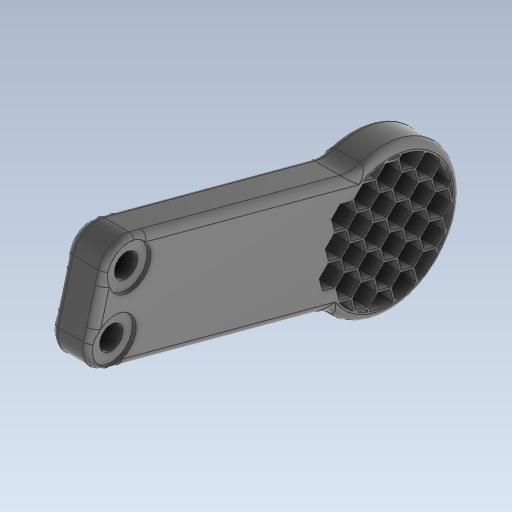
# Autodesk Inventor part: RearBumper
Saved by Autodesk Inventor 2020.4 (Build 244396000, 396)
## iProperties
Part Number: RearBumper
Material: PC/ABS プラスチック
Document SubType Name: Modeling
Designer: Masato Kubotera
Density: 0.357273 g/cm^3
Appearance: 滑らか - 黒
Description: TPU
Author: Masato Kubotera
Autodesk Inventor part; units mm, degrees
(part 1 of 2)
ref_plane "YZ Plane" through (0, 0, 0) normal (1, 0, 0) x (0, 1, 0)
ref_plane "XZ Plane" through (0, 0, 0) normal (0, 1, 0) x (-1, 0, 0)
ref_plane "XY Plane" through (0, 0, 0) normal (0, 0, 1) x (1, 0, 0)
derived "Trunk_basis.ipt"
sketch "スケッチ1" plane through (0, 0, 0) normal (0, 1, 0) x (-1, 0, 0)
  line L0 (0, 22) -> (0, -142.9) construction
  circle A0 centre (5, 0) radius 10.5 construction
  line L1 (-7, 16) -> (36, 16) construction
  line L2 (36, 16) -> (36, -16) construction
  line L3 (36, -16) -> (-7, -16) construction
  line L4 (-7, -16) -> (-7, 16) construction
  line L5 (-7, 16) -> (36, -16) construction
  line L6 (36, 16) -> (-7, -16) construction
  line L7 (33, 13.5) -> (6, 13.5) construction
  line L8 (6, 13.5) -> (6, -13.5) construction
  line L9 (6, -13.5) -> (33, -13.5) construction
  line L10 (33, -13.5) -> (33, 13.5) construction
  line L11 (33, 13.5) -> (6, -13.5) construction
  line L12 (6, 13.5) -> (33, -13.5) construction
  line L13 (-7, 0) -> (36, 0) construction
  arc A1 (5, 16) -> (-7, 10.583005) centre (5, 0) ccw construction
  line L14 (43.75, -16.25) -> (5, -16.25)
  line L15 (5, 16.25) -> (43.75, 16.25)
  line L16 (44.75, 15.25) -> (44.75, -15.25)
  arc A2 (5, 16.25) -> (-6.737613, 11.237924) centre (5, 0) ccw
  arc A3 (-6.737613, 11.237924) -> (-7.25, 9.917415) centre (-6.271109, 10.297247) ccw
  circle A4 centre (6, 13.5) radius 1.35
  line L17 (19.5, 13.5) -> (19.5, -13.5) construction
  circle A5 centre (33, 13.5) radius 1.35
  line L18 (-15, 22) -> (-20, 17)
  line L19 (-20, 17) -> (-20, -19)
  line L20 (-20, -19) -> (-28.5, -27.5)
  line L21 (-28.5, -27.5) -> (-28.5, -103)
  line L22 (57.5, -22.5) -> (57.5, 17)
  line L23 (57.5, 17) -> (52.5, 22)
  line L24 (52.5, 22) -> (-15, 22)
  line L25 (-35.55968, -116.552914) -> (-28.5, -142.9)
  line L26 (-16, -139) -> (-16, -94) construction
  line L27 (-7.5, -140.484924) -> (-7.5, -142.9)
  line L28 (-7.5, -142.9) -> (7.5, -142.9)
  line L29 (7.5, -140.484924) -> (7.5, -142.9)
  arc A6 (-7.5, -140.484924) -> (-8.984924, -139) centre (-8.242462, -139.742462) ccw
  line L30 (-17.5, -138.995456) -> (-17.5, -133) construction
  line L31 (-19, -133) -> (-16, -133) construction
  line L32 (-19, -133) -> (-19, -139) construction
  line L33 (-16, -133) -> (-16, -139) construction
  line L34 (-15, 22) -> (-10, 22) construction
  line L35 (-10, 22) -> (-10, -22) construction
  line L36 (-10, -22) -> (-15, -22) construction
  line L37 (-15, -22) -> (-15, 22) construction
  line L38 (-15, 22) -> (-10, -22) construction
  line L39 (-10, 22) -> (-15, -22) construction
  line L40 (-12.5, 22) -> (-12.5, -22) construction
  line L41 (-10, 0) -> (-15, 0) construction
  circle A7 centre (-12.5, 17.75) radius 1.6
  line L42 (-15, 10) -> (-12.5, 10) construction
  line L43 (-12.5, 10) -> (-12.5, -10) construction
  line L44 (-12.5, -10) -> (-15, -10) construction
  line L45 (-15, -10) -> (-15, 10) construction
  line L46 (-15, 10) -> (-12.5, -10) construction
  line L47 (-12.5, 10) -> (-15, -10) construction
  line L48 (-12.25, 10.25) -> (-15.25, 10.25)
  line L49 (-15.25, 8.15) -> (-15.25, -8.15)
  line L50 (-15.25, -10.25) -> (-12.25, -10.25)
  line L51 (-12.25, -8.15) -> (-12.25, 8.15)
  line L52 (-12.25, 10.25) -> (-15.25, -10.25) construction
  line L53 (-15.25, 10.25) -> (-12.25, -10.25) construction
  arc A8 (-15.25, 10.25) -> (-15.25, 8.15) centre (-15.25, 9.2) ccw
  line L54 (-13.75, 10) -> (-13.75, -10) construction
  arc A9 (-12.25, 8.15) -> (-12.25, 10.25) centre (-12.25, 9.2) ccw
  circle A10 centre (-12.5, -17.75) radius 1.6
  arc A11 (-15.25, -8.15) -> (-15.25, -10.25) centre (-15.25, -9.2) ccw
  arc A12 (-12.25, -10.25) -> (-12.25, -8.15) centre (-12.25, -9.2) ccw
  line L55 (36, 14.4) -> (44.5, 14.4) construction
  line L56 (44.5, 14.4) -> (44.5, -14.4) construction
  line L57 (36, -14.4) -> (44.5, -14.4) construction
  line L58 (49.95, 7.95) -> (49.95, -7.95)
  line L59 (52.5, 0) -> (47.5, 0) construction
  line L60 (47.5, 22) -> (52.5, 22) construction
  line L61 (52.55, -7.95) -> (52.55, 7.95)
  line L62 (51.25, 10) -> (51.25, -10) construction
  line L63 (52.5, 10) -> (50, -10) construction
  line L64 (52.5, -10) -> (50, -10) construction
  line L65 (52.5, 10) -> (52.5, -10) construction
  line L66 (50, 10) -> (52.5, -10) construction
  line L67 (49.95, -10.05) -> (52.55, -10.05)
  line L68 (49.95, 10.05) -> (52.55, -10.05) construction
  line L69 (52.55, 10.05) -> (49.95, -10.05) construction
  line L70 (52.5, -22) -> (47.5, -22) construction
  line L71 (47.5, 22) -> (52.5, -22) construction
  line L72 (52.5, 22) -> (52.5, -22) construction
  line L73 (52.5, 22) -> (47.5, -22) construction
  line L74 (50, 22) -> (50, -22) construction
  line L75 (47.5, -22) -> (47.5, 22) construction
  circle A13 centre (50, -17.75) radius 1.6
  arc A14 (52.55, -10.05) -> (52.55, -7.95) centre (52.55, -9) ccw
  line L76 (50, -10) -> (50, 10) construction
  arc A15 (49.95, -7.95) -> (49.95, -10.05) centre (49.95, -9) ccw
  arc A16 (49.95, 10.05) -> (49.95, 7.95) centre (49.95, 9) ccw
  arc A17 (52.55, 7.95) -> (52.55, 10.05) centre (52.55, 9) ccw
  line L77 (50, 10) -> (52.5, 10) construction
  line L78 (52.55, 10.05) -> (49.95, 10.05)
  circle A18 centre (50, 17.75) radius 1.6
  circle A19 centre (5, 0) radius 16 construction
  arc A20 (-6.737613, -11.237924) -> (5, -16.25) centre (5, 0) ccw
  arc A21 (-7.25, -9.917415) -> (-6.737613, -11.237924) centre (-6.271109, -10.297247) ccw
  line L79 (-7.25, -9.917415) -> (-7.25, 9.917415)
  line L80 (17.5, -138.995456) -> (17.5, -133) construction
  line L81 (19, -133) -> (19, -139) construction
  line L82 (16, -133) -> (16, -139) construction
  line L83 (19, -133) -> (16, -133) construction
  circle A22 centre (6, -13.5) radius 1.35
  circle A23 centre (33, -13.5) radius 1.35
  line L84 (-25.5, -142.9) -> (-7.5, -142.9) construction
  line L85 (25.5, -142.9) -> (7.5, -142.9) construction
  line L86 (-23.5, -22.5) -> (57.5, -22.5) construction
  line L87 (57.5, -22.5) -> (57.5, -103)
  circle A24 centre (-13.5, -55) radius 1.75
  line L88 (-16.5, -59) -> (45.5, -59)
  line L89 (47.5, -61) -> (47.5, -88)
  line L90 (45.5, -90) -> (-16.5, -90)
  line L91 (-18.5, -88) -> (-18.5, -61)
  line L92 (-18.5, -59) -> (47.5, -90) construction
  line L93 (47.5, -59) -> (-18.5, -90) construction
  line L94 (-16.5, -27.5) -> (45.5, -27.5)
  line L95 (47.5, -29.5) -> (47.5, -49)
  line L96 (45.5, -51) -> (-16.5, -51)
  line L97 (-18.5, -49) -> (-18.5, -29.5)
  line L98 (-18.5, -27.5) -> (47.5, -51) construction
  line L99 (47.5, -27.5) -> (-18.5, -51) construction
  line L100 (-23.5, -108) -> (-28.5, -103)
  circle A25 centre (-20.541452, -102) radius 1.6
  line L101 (-25.722674, -96) -> (25.722674, -96)
  line L102 (25.722674, -96) -> (34.960278, -112)
  line L103 (35.55968, -116.552914) -> (28.5, -142.9)
  line L104 (-25.722674, -96) -> (-34.960278, -112)
  line L105 (57.5, -103) -> (52.5, -108)
  arc A26 (-16.5, -27.5) -> (-18.5, -29.5) centre (-16.5, -29.5) ccw
  arc A27 (-18.5, -49) -> (-16.5, -51) centre (-16.5, -49) ccw
  arc A28 (45.5, -51) -> (47.5, -49) centre (45.5, -49) ccw
  arc A29 (47.5, -29.5) -> (45.5, -27.5) centre (45.5, -29.5) ccw
  arc A30 (-16.5, -59) -> (-18.5, -61) centre (-16.5, -61) ccw
  arc A31 (-18.5, -88) -> (-16.5, -90) centre (-16.5, -88) ccw
  arc A32 (45.5, -90) -> (47.5, -88) centre (45.5, -88) ccw
  arc A33 (47.5, -61) -> (45.5, -59) centre (45.5, -61) ccw
  line L106 (-23.5, -108) -> (52.5, -108)
  line L107 (-25.5, -139) -> (-25.5, -142.9)
  line L108 (-25.5, -142.9) -> (-28.5, -142.9)
  line L109 (-17.981292, -99.384327) -> (-16.996132, -101.090673)
  line L110 (-16.996132, -102.909327) -> (-17.981292, -104.615673)
  line L111 (-19.556292, -105.525) -> (-21.526612, -105.525)
  line L112 (-23.101612, -104.615673) -> (-24.086771, -102.909327)
  line L113 (-24.086771, -101.090673) -> (-23.101612, -99.384327)
  line L114 (-21.526612, -98.475) -> (-19.556292, -98.475)
  line L115 (-16, -94) -> (16, -94) construction
  arc A34 (-24.086771, -101.090673) -> (-24.086771, -102.909327) centre (-23.561771, -102) ccw
  arc A35 (-23.101612, -104.615673) -> (-21.526612, -105.525) centre (-22.051612, -104.615673) ccw
  arc A36 (-19.556292, -105.525) -> (-17.981292, -104.615673) centre (-19.031292, -104.615673) ccw
  arc A37 (-16.996132, -102.909327) -> (-16.996132, -101.090673) centre (-17.521132, -102) ccw
  arc A38 (-17.981292, -99.384327) -> (-19.556292, -98.475) centre (-19.031292, -99.384327) ccw
  arc A39 (-21.526612, -98.475) -> (-23.101612, -99.384327) centre (-22.051612, -99.384327) ccw
  line L116 (16, -139) -> (16, -94) construction
  line L117 (16, -94) -> (-16, -94) construction
  line L118 (-25.5, -139) -> (-8.984924, -139)
  line L119 (25.5, -142.9) -> (28.5, -142.9)
  arc A40 (8.984924, -139) -> (7.5, -140.484924) centre (8.242462, -139.742462) ccw
  circle A41 centre (29.764125, -115) radius 1.25
  line L120 (33.489128, -124.280321) -> (21.898018, -121.174492) construction
  line L121 (29.764125, -115) -> (25.623021, -130.454813) construction
  circle A42 centre (29.764125, -115) radius 6 construction
  circle A43 centre (-20.541452, -102) radius 6 construction
  line L122 (1.931852, -109.482362) -> (7.558785, -130.482362)
  line L123 (5.626933, -133) -> (-5.626933, -133)
  line L124 (5.315082, -110.517638) -> (10.942015, -131.517638)
  line L125 (12.873866, -133) -> (17.194729, -133)
  line L126 (19.126581, -131.517638) -> (24.753514, -110.517638)
  line L127 (22.821662, -108) -> (7.246933, -108)
  circle A44 centre (25.623021, -130.454813) radius 1.25
  circle A45 centre (25.623021, -130.454813) radius 6 construction
  line L128 (-1.931852, -109.482362) -> (-7.558785, -130.482362)
  arc A46 (1.931852, -109.482362) -> (-1.931852, -109.482362) centre (0, -110) ccw
  arc A47 (-7.558785, -130.482362) -> (-5.626933, -133) centre (-5.626933, -131) ccw
  arc A48 (5.626933, -133) -> (7.558785, -130.482362) centre (5.626933, -131) ccw
  arc A49 (7.246933, -108) -> (5.315082, -110.517638) centre (7.246933, -110) ccw
  arc A50 (24.753514, -110.517638) -> (22.821662, -108) centre (22.821662, -110) ccw
  arc A51 (17.194729, -133) -> (19.126581, -131.517638) centre (17.194729, -131) ccw
  arc A52 (10.942015, -131.517638) -> (12.873866, -133) centre (12.873866, -131) ccw
  arc A53 (-5.315082, -110.517638) -> (-7.246933, -108) centre (-7.246933, -110) ccw
  line L129 (-22.821662, -108) -> (-7.246933, -108)
  line L130 (-5.315082, -110.517638) -> (-10.942015, -131.517638)
  arc A54 (-22.821662, -108) -> (-24.753514, -110.517638) centre (-22.821662, -110) ccw
  line L131 (-19.126581, -131.517638) -> (-24.753514, -110.517638)
  arc A55 (-19.126581, -131.517638) -> (-17.194729, -133) centre (-17.194729, -131) ccw
  line L132 (-12.873866, -133) -> (-17.194729, -133)
  arc A56 (-12.873866, -133) -> (-10.942015, -131.517638) centre (-12.873866, -131) ccw
  circle A57 centre (-29.764125, -115) radius 1.25
  circle A58 centre (-25.623021, -130.454813) radius 1.25
  arc A59 (35.55968, -116.552914) -> (34.960278, -112) centre (29.764125, -115) ccw
  arc A60 (-34.960278, -112) -> (-35.55968, -116.552914) centre (-29.764125, -115) ccw
  arc A61 (-24.015076, -139) -> (-25.5, -140.484924) centre (-24.757538, -139.742462) ccw
  line L133 (25.5, -139) -> (25.5, -142.9)
  arc A62 (25.5, -140.484924) -> (24.015076, -139) centre (24.757538, -139.742462) ccw
  line L134 (25.5, -139) -> (8.984924, -139)
  line L135 (21.526612, -98.475) -> (19.556292, -98.475)
  line L136 (16.996132, -102.909327) -> (17.981292, -104.615673)
  arc A63 (21.526612, -105.525) -> (23.101612, -104.615673) centre (22.051612, -104.615673) ccw
  circle A64 centre (20.541452, -102) radius 1.6
  line L137 (24.086771, -101.090673) -> (23.101612, -99.384327)
  arc A65 (24.086771, -102.909327) -> (24.086771, -101.090673) centre (23.561771, -102) ccw
  line L138 (23.101612, -104.615673) -> (24.086771, -102.909327)
  arc A66 (23.101612, -99.384327) -> (21.526612, -98.475) centre (22.051612, -99.384327) ccw
  line L139 (19.556292, -105.525) -> (21.526612, -105.525)
  arc A67 (19.556292, -98.475) -> (17.981292, -99.384327) centre (19.031292, -99.384327) ccw
  arc A68 (17.981292, -104.615673) -> (19.556292, -105.525) centre (19.031292, -104.615673) ccw
  line L140 (17.981292, -99.384327) -> (16.996132, -101.090673)
  arc A69 (16.996132, -101.090673) -> (16.996132, -102.909327) centre (17.521132, -102) ccw
  line L141 (16, -139) -> (16, -94) construction
  circle A70 centre (20.541452, -102) radius 6 construction
  arc A71 (29.504521, -117.544512) -> (31.261205, -117.073809) centre (30.246983, -116.802049) ccw construction
  line L142 (31.837935, -116.49708) -> (31.261205, -117.073809) construction
  line L143 (29.504521, -117.544512) -> (28.716694, -117.333414) construction
  arc A72 (27.430712, -116.047432) -> (28.716694, -117.333414) centre (28.444934, -116.319192) ccw construction
  line L144 (27.430712, -116.047432) -> (27.219614, -115.259604) construction
  line L145 (27.690316, -113.50292) -> (28.267046, -112.926191) construction
  arc A73 (30.02373, -112.455488) -> (28.267046, -112.926191) centre (29.281268, -113.197951) ccw construction
  arc A74 (27.690316, -113.50292) -> (27.219614, -115.259604) centre (27.962076, -114.517142) ccw construction
  line L146 (30.02373, -112.455488) -> (30.811557, -112.666586) construction
  arc A75 (31.837935, -116.49708) -> (32.308637, -114.740396) centre (31.566175, -115.482858) ccw construction
  arc A76 (32.097539, -113.952568) -> (30.811557, -112.666586) centre (31.083317, -113.680808) ccw construction
  line L147 (32.097539, -113.952568) -> (32.308637, -114.740396) construction
  line L148 (-20.541452, -102) -> (20.541452, -102) construction
  circle A77 centre (0, -102) radius 1.6
  line L149 (0.407809, -104.525) -> (-0.407809, -104.525)
  arc A78 (-0.407809, -99.475) -> (-1.982809, -100.384327) centre (-0.932809, -100.384327) ccw
  arc A79 (0.407809, -104.525) -> (1.982809, -103.615673) centre (0.932809, -103.615673) ccw
  line L150 (2.390619, -102.909327) -> (1.982809, -103.615673)
  line L151 (-0.407809, -99.475) -> (0.407809, -99.475)
  arc A80 (1.982809, -100.384327) -> (0.407809, -99.475) centre (0.932809, -100.384327) ccw
  line L152 (1.982809, -100.384327) -> (2.390619, -101.090673)
  arc A81 (2.390619, -102.909327) -> (2.390619, -101.090673) centre (1.865619, -102) ccw
  line L153 (-2.390619, -101.090673) -> (-1.982809, -100.384327)
  arc A82 (-2.390619, -101.090673) -> (-2.390619, -102.909327) centre (-1.865619, -102) ccw
  line L154 (-1.982809, -103.615673) -> (-2.390619, -102.909327)
  arc A83 (-1.982809, -103.615673) -> (-0.407809, -104.525) centre (-0.932809, -103.615673) ccw
  circle A84 centre (0, -102) radius 1.25
  arc A85 (44.75, 15.25) -> (43.75, 16.25) centre (43.75, 15.25) ccw
  arc A86 (43.75, -16.25) -> (44.75, -15.25) centre (43.75, -15.25) ccw
  point P0 (0, 0)
  point P1 (14.5, 0)
  point P2 (19.5, 0)
  point P3 (44.75, 16.25)
  point P4 (-7.25, 10.677078)
  point P5 (19.5, 0)
  point P6 (-12.5, 0)
  point P7 (-13.75, 0)
  point P8 (44.75, 14.4)
  point P9 (44.75, -14.4)
  point P10 (51.25, 0)
  point P11 (50, 0)
  point P12 (44.75, -16.25)
  point P13 (14.5, -74.5)
  point P14 (14.5, -39.25)
  point P15 (-18.506292, -98.475)
  point P16 (-16.471132, -102)
  point P17 (-18.506292, -105.525)
  point P18 (-22.576612, -105.525)
  point P19 (-22.576612, -98.475)
  point P20 (-24.611771, -102)
  point P21 (-22.576612, -105.525)
  point P22 (-18.506292, -105.525)
  point P23 (-16.471132, -102)
  point P24 (-18.506292, -98.475)
  point P25 (-22.576612, -98.475)
  point P26 (27.693573, -122.727407)
  point P27 (0, -102.272593)
  point P28 (0, -133)
  point P29 (-7.5, -139)
  point P30 (-22.576612, -98.475)
  point P31 (18.506292, -98.475)
  point P32 (18.506292, -98.475)
  point P33 (22.576612, -105.525)
  point P34 (22.576612, -105.525)
  point P35 (24.611771, -102)
  point P36 (22.576612, -98.475)
  point P37 (22.576612, -98.475)
  point P38 (22.576612, -98.475)
  point P39 (18.506292, -105.525)
  point P40 (16.471132, -102)
  point P41 (16.471132, -102)
  point P42 (18.506292, -105.525)
  point P43 (29.764125, -115)
  point P44 (29.764125, -115)
  point P45 (30.518743, -117.816272)
  point P46 (30.518743, -117.816272)
  point P47 (27.702472, -117.061654)
  point P48 (27.702472, -117.061654)
  point P49 (31.825779, -112.938346)
  point P50 (26.947854, -114.245382)
  point P51 (29.009508, -112.183728)
  point P52 (29.009508, -112.183728)
  point P53 (31.825779, -112.938346)
  point P54 (29.009508, -112.183728)
  point P55 (32.580397, -115.754618)
  point P56 (-1.457809, -99.475)
  point P57 (-1.457809, -99.475)
  point P58 (-1.457809, -99.475)
  point P59 (1.457809, -104.525)
  point P60 (1.457809, -99.475)
  point P61 (1.457809, -99.475)
  point P62 (2.915619, -102)
  point P63 (-2.915619, -102)
  point P64 (-1.457809, -104.525)
  point P65 (-1.457809, -104.525)
sketch "スケッチ2" plane through (0, 0, 0) normal (0, 1, 0) x (-1, 0, 0)
  circle A0 centre (29.764125, -115) radius 1.25
  circle A1 centre (25.623021, -130.454813) radius 1.25
  circle A2 centre (29.764125, -115) radius 3.25
  arc A3 (31.575859, -108.238519) -> (23.002645, -113.188267) centre (29.764125, -115) ccw
  line L0 (31.575859, -108.238519) -> (93.882286, -124.933476)
  line L1 (33.489128, -124.280321) -> (21.898018, -121.174492) construction
  circle A4 centre (25.623021, -130.454813) radius 3.25
  arc A5 (18.86154, -128.64308) -> (23.811287, -137.216294) centre (25.623021, -130.454813) ccw
  line L2 (23.811287, -137.216294) -> (86.117714, -153.911251)
  line L3 (0, 22) -> (0, -142.9) construction
  line L4 (23.002645, -113.188267) -> (18.86154, -128.64308)
  circle A6 centre (29.764125, -115) radius 6
  circle A7 centre (25.623021, -130.454813) radius 6
  arc A8 (86.117714, -153.911251) -> (93.882286, -124.933476) centre (102.777998, -142.846218) ccw
  arc A9 (86.117714, -153.911251) -> (93.882286, -124.933476) centre (90, -139.422363) ccw
  arc A10 (88.527846, -153.004129) -> (95.51596, -126.924132) centre (102.777998, -142.846218) ccw
  line L5 (91.324519, -139.777267) -> (88.875029, -142.226757)
  line L6 (88.875029, -142.226757) -> (85.528964, -141.330181)
  line L7 (85.528964, -141.330181) -> (84.632388, -137.984116)
  line L8 (84.632388, -137.984116) -> (87.081878, -135.534626)
  line L9 (87.081878, -135.534626) -> (90.427943, -136.431202)
  line L10 (90.427943, -136.431202) -> (91.324519, -139.777267)
  line L11 (85.080676, -139.657149) -> (90.876231, -138.104235) construction
  line L12 (85.857133, -136.759371) -> (90.099774, -141.002012) construction
  line L13 (84.632388, -137.984116) -> (91.324519, -139.777267) construction
  line L14 (91.007499, -136.27591) -> (93.456988, -133.826421)
  line L15 (91.904074, -139.621976) -> (91.007499, -136.27591)
  line L16 (95.250139, -140.518551) -> (91.904074, -139.621976)
  line L17 (97.699629, -138.069061) -> (95.250139, -140.518551)
  line L18 (96.803054, -134.722996) -> (97.699629, -138.069061)
  line L19 (93.456988, -133.826421) -> (96.803054, -134.722996)
  line L20 (89.299293, -142.651021) -> (91.748783, -140.201531)
  line L21 (90.195868, -145.997086) -> (89.299293, -142.651021)
  line L22 (93.541934, -146.893662) -> (90.195868, -145.997086)
  line L23 (95.991423, -144.444172) -> (93.541934, -146.893662)
  line L24 (95.094848, -141.098107) -> (95.991423, -144.444172)
  line L25 (91.748783, -140.201531) -> (95.094848, -141.098107)
  line L26 (98.123893, -138.493325) -> (101.469958, -139.389901)
  line L27 (95.674403, -140.942815) -> (98.123893, -138.493325)
  line L28 (96.570979, -144.28888) -> (95.674403, -140.942815)
  line L29 (99.917044, -145.185456) -> (96.570979, -144.28888)
  line L30 (102.366534, -142.735966) -> (99.917044, -145.185456)
  line L31 (101.469958, -139.389901) -> (102.366534, -142.735966)
  line L32 (102.790798, -143.16023) -> (106.136863, -144.056806)
  line L33 (100.341308, -145.60972) -> (102.790798, -143.16023)
  line L34 (101.237884, -148.955785) -> (100.341308, -145.60972)
  line L35 (104.583949, -149.852361) -> (101.237884, -148.955785)
  line L36 (107.033439, -147.402871) -> (104.583949, -149.852361)
  line L37 (106.136863, -144.056806) -> (107.033439, -147.402871)
  line L38 (106.292155, -143.47725) -> (102.946089, -142.580675)
  line L39 (108.741644, -141.02776) -> (106.292155, -143.47725)
  line L40 (107.845069, -137.681695) -> (108.741644, -141.02776)
  line L41 (104.499004, -136.78512) -> (107.845069, -137.681695)
  line L42 (102.049514, -139.23461) -> (104.499004, -136.78512)
  line L43 (102.946089, -142.580675) -> (102.049514, -139.23461)
  line L44 (109.165908, -141.452025) -> (112.511974, -142.3486)
  line L45 (106.716419, -143.901514) -> (109.165908, -141.452025)
  line L46 (107.612994, -147.247579) -> (106.716419, -143.901514)
  line L47 (110.959059, -148.144155) -> (107.612994, -147.247579)
  line L48 (113.408549, -145.694665) -> (110.959059, -148.144155)
  line L49 (112.511974, -142.3486) -> (113.408549, -145.694665)
  line L50 (113.832813, -146.118929) -> (117.178878, -147.015505)
  line L51 (111.383323, -148.568419) -> (113.832813, -146.118929)
  line L52 (112.279899, -151.914484) -> (111.383323, -148.568419)
  line L53 (115.625964, -152.81106) -> (112.279899, -151.914484)
  line L54 (118.075454, -150.36157) -> (115.625964, -152.81106)
  line L55 (117.178878, -147.015505) -> (118.075454, -150.36157)
  line L56 (117.33417, -146.435949) -> (113.988105, -145.539374)
  line L57 (119.78366, -143.98646) -> (117.33417, -146.435949)
  line L58 (118.887084, -140.640394) -> (119.78366, -143.98646)
  line L59 (115.541019, -139.743819) -> (118.887084, -140.640394)
  line L60 (113.091529, -142.193309) -> (115.541019, -139.743819)
  line L61 (113.988105, -145.539374) -> (113.091529, -142.193309)
  line L62 (120.207924, -144.410724) -> (123.553989, -145.307299)
  line L63 (117.758434, -146.860213) -> (120.207924, -144.410724)
  line L64 (118.655009, -150.206279) -> (117.758434, -146.860213)
  line L65 (122.001075, -151.102854) -> (118.655009, -150.206279)
  line L66 (124.450564, -148.653364) -> (122.001075, -151.102854)
  line L67 (123.553989, -145.307299) -> (124.450564, -148.653364)
  line L68 (124.874828, -149.077628) -> (128.220894, -149.974204)
  line L69 (122.425339, -151.527118) -> (124.874828, -149.077628)
  line L70 (123.321914, -154.873183) -> (122.425339, -151.527118)
  line L71 (126.667979, -155.769759) -> (123.321914, -154.873183)
  line L72 (129.117469, -153.320269) -> (126.667979, -155.769759)
  line L73 (128.220894, -149.974204) -> (129.117469, -153.320269)
  line L74 (128.376185, -149.394648) -> (125.03012, -148.498073)
  line L75 (130.825675, -146.945159) -> (128.376185, -149.394648)
  line L76 (129.929099, -143.599093) -> (130.825675, -146.945159)
  line L77 (126.583034, -142.702518) -> (129.929099, -143.599093)
  line L78 (124.133544, -145.152008) -> (126.583034, -142.702518)
  line L79 (125.03012, -148.498073) -> (124.133544, -145.152008)
  line L80 (90.583235, -135.851646) -> (87.237169, -134.955071)
  line L81 (87.237169, -134.955071) -> (86.340594, -131.609006)
  line L82 (86.340594, -131.609006) -> (88.790084, -129.159516)
  line L83 (88.790084, -129.159516) -> (92.136149, -130.056091)
  line L84 (92.136149, -130.056091) -> (93.032724, -133.402157)
  line L85 (93.032724, -133.402157) -> (90.583235, -135.851646)
  line L86 (92.715704, -129.9008) -> (95.165194, -127.45131)
  line L87 (93.61228, -133.246865) -> (92.715704, -129.9008)
  line L88 (96.958345, -134.143441) -> (93.61228, -133.246865)
  line L89 (99.407835, -131.693951) -> (96.958345, -134.143441)
  line L90 (98.511259, -128.347886) -> (99.407835, -131.693951)
  line L91 (95.165194, -127.45131) -> (98.511259, -128.347886)
  line L92 (97.382609, -134.567705) -> (99.832099, -132.118215)
  line L93 (99.832099, -132.118215) -> (103.178164, -133.014791)
  line L94 (98.279185, -137.91377) -> (97.382609, -134.567705)
  line L95 (101.62525, -138.810345) -> (98.279185, -137.91377)
  line L96 (104.07474, -136.360856) -> (101.62525, -138.810345)
  line L97 (103.178164, -133.014791) -> (104.07474, -136.360856)
  line L98 (104.654295, -136.205564) -> (103.75772, -132.859499)
  line L99 (103.75772, -132.859499) -> (106.207209, -130.410009)
  line L100 (106.207209, -130.410009) -> (109.553275, -131.306585)
  line L101 (109.553275, -131.306585) -> (110.44985, -134.65265)
  line L102 (110.44985, -134.65265) -> (108.00036, -137.10214)
  line L103 (108.00036, -137.10214) -> (104.654295, -136.205564)
  line L104 (108.424624, -137.526404) -> (110.874114, -135.076914)
  line L105 (110.874114, -135.076914) -> (114.220179, -135.97349)
  line L106 (114.220179, -135.97349) -> (115.116755, -139.319555)
  line L107 (115.116755, -139.319555) -> (112.667265, -141.769045)
  line L108 (112.667265, -141.769045) -> (109.3212, -140.872469)
  line L109 (109.3212, -140.872469) -> (108.424624, -137.526404)
  line L110 (115.69631, -139.164263) -> (114.799735, -135.818198)
  line L111 (114.799735, -135.818198) -> (117.249225, -133.368708)
  line L112 (117.249225, -133.368708) -> (120.59529, -134.265284)
  line L113 (120.59529, -134.265284) -> (121.491865, -137.611349)
  line L114 (121.491865, -137.611349) -> (119.042376, -140.060839)
  line L115 (119.042376, -140.060839) -> (115.69631, -139.164263)
  line L116 (120.363215, -143.831168) -> (119.46664, -140.485103)
  line L117 (119.46664, -140.485103) -> (121.916129, -138.035613)
  line L118 (121.916129, -138.035613) -> (125.262195, -138.932189)
  line L119 (125.262195, -138.932189) -> (126.15877, -142.278254)
  line L120 (126.15877, -142.278254) -> (123.70928, -144.727744)
  line L121 (123.70928, -144.727744) -> (120.363215, -143.831168)
  line L122 (130.084391, -143.019538) -> (126.738325, -142.122962)
  line L123 (126.738325, -142.122962) -> (125.84175, -138.776897)
  line L124 (125.84175, -138.776897) -> (128.29124, -136.327407)
  line L125 (128.29124, -136.327407) -> (131.637305, -137.223983)
  line L126 (131.637305, -137.223983) -> (132.53388, -140.570048)
  line L127 (132.53388, -140.570048) -> (130.084391, -143.019538)
  line L128 (92.29144, -129.476536) -> (88.945375, -128.57996)
  line L129 (88.945375, -128.57996) -> (88.0488, -125.233895)
  line L130 (88.0488, -125.233895) -> (90.498289, -122.784406)
  line L131 (90.498289, -122.784406) -> (93.844355, -123.680981)
  line L132 (93.844355, -123.680981) -> (94.74093, -127.027046)
  line L133 (94.74093, -127.027046) -> (92.29144, -129.476536)
  line L134 (94.42391, -123.52569) -> (96.8734, -121.0762)
  line L135 (95.320486, -126.871755) -> (94.42391, -123.52569)
  line L136 (98.666551, -127.76833) -> (95.320486, -126.871755)
  line L137 (101.116041, -125.318841) -> (98.666551, -127.76833)
  line L138 (100.219465, -121.972775) -> (101.116041, -125.318841)
  line L139 (96.8734, -121.0762) -> (100.219465, -121.972775)
  line L140 (99.090815, -128.192594) -> (101.540305, -125.743105)
  line L141 (101.540305, -125.743105) -> (104.88637, -126.63968)
  line L142 (99.98739, -131.53866) -> (99.090815, -128.192594)
  line L143 (103.333456, -132.435235) -> (99.98739, -131.53866)
  line L144 (105.782945, -129.985745) -> (103.333456, -132.435235)
  line L145 (104.88637, -126.63968) -> (105.782945, -129.985745)
  line L146 (106.362501, -129.830454) -> (105.465925, -126.484389)
  line L147 (105.465925, -126.484389) -> (107.915415, -124.034899)
  line L148 (107.915415, -124.034899) -> (111.26148, -124.931474)
  line L149 (111.26148, -124.931474) -> (112.158056, -128.27754)
  line L150 (112.158056, -128.27754) -> (109.708566, -130.727029)
  line L151 (109.708566, -130.727029) -> (106.362501, -129.830454)
  line L152 (110.13283, -131.151293) -> (112.58232, -128.701804)
  line L153 (112.58232, -128.701804) -> (115.928385, -129.598379)
  line L154 (115.928385, -129.598379) -> (116.82496, -132.944444)
  line L155 (116.82496, -132.944444) -> (114.375471, -135.393934)
  line L156 (114.375471, -135.393934) -> (111.029406, -134.497359)
  line L157 (111.029406, -134.497359) -> (110.13283, -131.151293)
  line L158 (117.404516, -132.789153) -> (116.507941, -129.443088)
  line L159 (116.507941, -129.443088) -> (118.95743, -126.993598)
  line L160 (118.95743, -126.993598) -> (122.303495, -127.890173)
  line L161 (122.303495, -127.890173) -> (123.200071, -131.236239)
  line L162 (123.200071, -131.236239) -> (120.750581, -133.685728)
  line L163 (120.750581, -133.685728) -> (117.404516, -132.789153)
  line L164 (122.071421, -137.456058) -> (121.174845, -134.109992)
  line L165 (121.174845, -134.109992) -> (123.624335, -131.660503)
  line L166 (123.624335, -131.660503) -> (126.9704, -132.557078)
  line L167 (126.9704, -132.557078) -> (127.866976, -135.903143)
  line L168 (127.866976, -135.903143) -> (125.417486, -138.352633)
  line L169 (125.417486, -138.352633) -> (122.071421, -137.456058)
  line L170 (131.792596, -136.644427) -> (128.446531, -135.747852)
  line L171 (128.446531, -135.747852) -> (127.549956, -132.401787)
  line L172 (127.549956, -132.401787) -> (129.999445, -129.952297)
  line L173 (129.999445, -129.952297) -> (133.345511, -130.848872)
  line L174 (133.345511, -130.848872) -> (134.242086, -134.194938)
  line L175 (134.242086, -134.194938) -> (131.792596, -136.644427)
  line L176 (89.616313, -146.152378) -> (87.166823, -148.601867)
  line L177 (88.719738, -142.806312) -> (89.616313, -146.152378)
  line L178 (85.373672, -141.909737) -> (88.719738, -142.806312)
  line L179 (82.924183, -144.359227) -> (85.373672, -141.909737)
  line L180 (83.820758, -147.705292) -> (82.924183, -144.359227)
  line L181 (87.166823, -148.601867) -> (83.820758, -147.705292)
  line L182 (87.591087, -149.026131) -> (90.040577, -146.576642)
  line L183 (90.040577, -146.576642) -> (93.386642, -147.473217)
  line L184 (93.386642, -147.473217) -> (94.283218, -150.819282)
  line L185 (94.283218, -150.819282) -> (91.833728, -153.268772)
  line L186 (91.833728, -153.268772) -> (88.487663, -152.372197)
  line L187 (88.487663, -152.372197) -> (87.591087, -149.026131)
  line L188 (98.633103, -151.98483) -> (101.082592, -149.535341)
  line L189 (99.529678, -155.330896) -> (98.633103, -151.98483)
  line L190 (100.658328, -149.111077) -> (98.208838, -151.560566)
  line L191 (98.208838, -151.560566) -> (94.862773, -150.663991)
  line L192 (94.862773, -150.663991) -> (93.966198, -147.317926)
  line L193 (93.966198, -147.317926) -> (96.415688, -144.868436)
  line L194 (96.415688, -144.868436) -> (99.761753, -145.765011)
  line L195 (99.761753, -145.765011) -> (100.658328, -149.111077)
  line L196 (101.082592, -149.535341) -> (104.428657, -150.431916)
  line L197 (104.428657, -150.431916) -> (105.325233, -153.777981)
  line L198 (105.325233, -153.777981) -> (102.875743, -156.227471)
  line L199 (102.875743, -156.227471) -> (99.529678, -155.330896)
  line L200 (109.250854, -154.519265) -> (105.904788, -153.62269)
  line L201 (105.904788, -153.62269) -> (105.008213, -150.276625)
  line L202 (105.008213, -150.276625) -> (107.457703, -147.827135)
  line L203 (107.457703, -147.827135) -> (110.803768, -148.72371)
  line L204 (110.803768, -148.72371) -> (111.700343, -152.069776)
  line L205 (111.700343, -152.069776) -> (109.250854, -154.519265)
  line L206 (112.124607, -152.49404) -> (115.470673, -153.390615)
  line L207 (109.675118, -154.943529) -> (112.124607, -152.49404)
  line L208 (110.571693, -158.289595) -> (109.675118, -154.943529)
  line L209 (113.917758, -159.18617) -> (110.571693, -158.289595)
  line L210 (116.367248, -156.73668) -> (113.917758, -159.18617)
  line L211 (115.470673, -153.390615) -> (116.367248, -156.73668)
  line L212 (122.742359, -155.028475) -> (120.292869, -157.477964)
  line L213 (120.292869, -157.477964) -> (116.946804, -156.581389)
  line L214 (116.050228, -153.235324) -> (118.499718, -150.785834)
  line L215 (116.946804, -156.581389) -> (116.050228, -153.235324)
  line L216 (118.499718, -150.785834) -> (121.845783, -151.68241)
  line L217 (121.845783, -151.68241) -> (122.742359, -155.028475)
  line L218 (120.717133, -157.902229) -> (123.166623, -155.452739)
  line L219 (123.166623, -155.452739) -> (126.512688, -156.349314)
  line L220 (126.512688, -156.349314) -> (127.409263, -159.695379)
  line L221 (127.409263, -159.695379) -> (124.959774, -162.144869)
  line L222 (124.959774, -162.144869) -> (121.613708, -161.248294)
  line L223 (121.613708, -161.248294) -> (120.717133, -157.902229)
  line L224 (87.908107, -152.527488) -> (85.458618, -154.976978)
  line L225 (87.011532, -149.181423) -> (87.908107, -152.527488)
  line L226 (83.665467, -148.284847) -> (87.011532, -149.181423)
  line L227 (81.215977, -150.734337) -> (83.665467, -148.284847)
  line L228 (82.112552, -154.080402) -> (81.215977, -150.734337)
  line L229 (85.458618, -154.976978) -> (82.112552, -154.080402)
  line L230 (85.882882, -155.401242) -> (88.332371, -152.951752)
  line L231 (88.332371, -152.951752) -> (91.678437, -153.848328)
  line L232 (91.678437, -153.848328) -> (92.575012, -157.194393)
  line L233 (92.575012, -157.194393) -> (90.125522, -159.643883)
  line L234 (90.125522, -159.643883) -> (86.779457, -158.747307)
  line L235 (86.779457, -158.747307) -> (85.882882, -155.401242)
  line L236 (96.924897, -158.359941) -> (99.374387, -155.910451)
  line L237 (97.821472, -161.706006) -> (96.924897, -158.359941)
  line L238 (98.950122, -155.486187) -> (96.500633, -157.935677)
  line L239 (96.500633, -157.935677) -> (93.154568, -157.039101)
  line L240 (93.154568, -157.039101) -> (92.257992, -153.693036)
  line L241 (92.257992, -153.693036) -> (94.707482, -151.243546)
  line L242 (94.707482, -151.243546) -> (98.053547, -152.140122)
  line L243 (98.053547, -152.140122) -> (98.950122, -155.486187)
  line L244 (99.374387, -155.910451) -> (102.720452, -156.807027)
  line L245 (102.720452, -156.807027) -> (103.617027, -160.153092)
  line L246 (103.617027, -160.153092) -> (101.167538, -162.602582)
  line L247 (101.167538, -162.602582) -> (97.821472, -161.706006)
  line L248 (107.542648, -160.894376) -> (104.196583, -159.9978)
  line L249 (104.196583, -159.9978) -> (103.300007, -156.651735)
  line L250 (103.300007, -156.651735) -> (105.749497, -154.202245)
  line L251 (105.749497, -154.202245) -> (109.095562, -155.098821)
  line L252 (109.095562, -155.098821) -> (109.992138, -158.444886)
  line L253 (109.992138, -158.444886) -> (107.542648, -160.894376)
  line L254 (110.416402, -158.86915) -> (113.762467, -159.765726)
  line L255 (107.966912, -161.31864) -> (110.416402, -158.86915)
  line L256 (108.863487, -164.664705) -> (107.966912, -161.31864)
  line L257 (112.209553, -165.561281) -> (108.863487, -164.664705)
  line L258 (114.659042, -163.111791) -> (112.209553, -165.561281)
  line L259 (113.762467, -159.765726) -> (114.659042, -163.111791)
  line L260 (121.034153, -161.403585) -> (118.584663, -163.853075)
  line L261 (118.584663, -163.853075) -> (115.238598, -162.956499)
  line L262 (114.342022, -159.610434) -> (116.791512, -157.160945)
  line L263 (115.238598, -162.956499) -> (114.342022, -159.610434)
  line L264 (116.791512, -157.160945) -> (120.137577, -158.05752)
  line L265 (120.137577, -158.05752) -> (121.034153, -161.403585)
  line L266 (119.008927, -164.277339) -> (121.458417, -161.827849)
  line L267 (121.458417, -161.827849) -> (124.804482, -162.724425)
  line L268 (124.804482, -162.724425) -> (125.701058, -166.07049)
  line L269 (125.701058, -166.07049) -> (123.251568, -168.51998)
  line L270 (123.251568, -168.51998) -> (119.905503, -167.623404)
  line L271 (119.905503, -167.623404) -> (119.008927, -164.277339)
  line L272 (86.199902, -158.902598) -> (83.750412, -161.352088)
  line L273 (85.303326, -155.556533) -> (86.199902, -158.902598)
  line L274 (81.957261, -154.659958) -> (85.303326, -155.556533)
  line L275 (79.507771, -157.109448) -> (81.957261, -154.659958)
  line L276 (80.404347, -160.455513) -> (79.507771, -157.109448)
  line L277 (83.750412, -161.352088) -> (80.404347, -160.455513)
  line L278 (84.174676, -161.776352) -> (86.624166, -159.326863)
  line L279 (86.624166, -159.326863) -> (89.970231, -160.223438)
  line L280 (89.970231, -160.223438) -> (90.866806, -163.569503)
  line L281 (90.866806, -163.569503) -> (88.417317, -166.018993)
  line L282 (88.417317, -166.018993) -> (85.071251, -165.122417)
  line L283 (85.071251, -165.122417) -> (84.174676, -161.776352)
  line L284 (95.216691, -164.735051) -> (97.666181, -162.285562)
  line L285 (96.113267, -168.081117) -> (95.216691, -164.735051)
  line L286 (97.241917, -161.861298) -> (94.792427, -164.310787)
  line L287 (94.792427, -164.310787) -> (91.446362, -163.414212)
  line L288 (91.446362, -163.414212) -> (90.549786, -160.068147)
  line L289 (90.549786, -160.068147) -> (92.999276, -157.618657)
  line L290 (92.999276, -157.618657) -> (96.345341, -158.515232)
  line L291 (96.345341, -158.515232) -> (97.241917, -161.861298)
  line L292 (97.666181, -162.285562) -> (101.012246, -163.182137)
  line L293 (101.012246, -163.182137) -> (101.908822, -166.528202)
  line L294 (101.908822, -166.528202) -> (99.459332, -168.977692)
  line L295 (99.459332, -168.977692) -> (96.113267, -168.081117)
  line L296 (105.834442, -167.269486) -> (102.488377, -166.372911)
  line L297 (102.488377, -166.372911) -> (101.591802, -163.026846)
  line L298 (101.591802, -163.026846) -> (104.041291, -160.577356)
  line L299 (104.041291, -160.577356) -> (107.387357, -161.473931)
  line L300 (107.387357, -161.473931) -> (108.283932, -164.819997)
  line L301 (108.283932, -164.819997) -> (105.834442, -167.269486)
  line L302 (108.708196, -165.244261) -> (112.054261, -166.140836)
  line L303 (106.258706, -167.69375) -> (108.708196, -165.244261)
  line L304 (107.155282, -171.039816) -> (106.258706, -167.69375)
  line L305 (110.501347, -171.936391) -> (107.155282, -171.039816)
  line L306 (112.950837, -169.486901) -> (110.501347, -171.936391)
  line L307 (112.054261, -166.140836) -> (112.950837, -169.486901)
  line L308 (119.325947, -167.778696) -> (116.876457, -170.228185)
  line L309 (116.876457, -170.228185) -> (113.530392, -169.33161)
  line L310 (112.633817, -165.985545) -> (115.083307, -163.536055)
  line L311 (113.530392, -169.33161) -> (112.633817, -165.985545)
  line L312 (115.083307, -163.536055) -> (118.429372, -164.43263)
  line L313 (118.429372, -164.43263) -> (119.325947, -167.778696)
  line L314 (117.300722, -170.652449) -> (119.750211, -168.20296)
  line L315 (119.750211, -168.20296) -> (123.096276, -169.099535)
  line L316 (123.096276, -169.099535) -> (123.992852, -172.4456)
  line L317 (123.992852, -172.4456) -> (121.543362, -174.89509)
  line L318 (121.543362, -174.89509) -> (118.197297, -173.998515)
  line L319 (118.197297, -173.998515) -> (117.300722, -170.652449)
  line L320 (93.999646, -123.101425) -> (90.653581, -122.20485)
  line L321 (90.653581, -122.20485) -> (89.757005, -118.858785)
  line L322 (89.757005, -118.858785) -> (92.206495, -116.409295)
  line L323 (92.206495, -116.409295) -> (95.55256, -117.305871)
  line L324 (95.55256, -117.305871) -> (96.449136, -120.651936)
  line L325 (96.449136, -120.651936) -> (93.999646, -123.101425)
  line L326 (96.132116, -117.150579) -> (98.581606, -114.701089)
  line L327 (97.028691, -120.496644) -> (96.132116, -117.150579)
  line L328 (100.374756, -121.39322) -> (97.028691, -120.496644)
  line L329 (102.824246, -118.94373) -> (100.374756, -121.39322)
  line L330 (101.927671, -115.597665) -> (102.824246, -118.94373)
  line L331 (98.581606, -114.701089) -> (101.927671, -115.597665)
  line L332 (100.799021, -121.817484) -> (103.24851, -119.367994)
  line L333 (103.24851, -119.367994) -> (106.594576, -120.26457)
  line L334 (101.695596, -125.163549) -> (100.799021, -121.817484)
  line L335 (105.041661, -126.060125) -> (101.695596, -125.163549)
  line L336 (107.491151, -123.610635) -> (105.041661, -126.060125)
  line L337 (106.594576, -120.26457) -> (107.491151, -123.610635)
  line L338 (108.070706, -123.455343) -> (107.174131, -120.109278)
  line L339 (107.174131, -120.109278) -> (109.623621, -117.659788)
  line L340 (109.623621, -117.659788) -> (112.969686, -118.556364)
  line L341 (112.969686, -118.556364) -> (113.866261, -121.902429)
  line L342 (113.866261, -121.902429) -> (111.416772, -124.351919)
  line L343 (111.416772, -124.351919) -> (108.070706, -123.455343)
  line L344 (111.841036, -124.776183) -> (114.290526, -122.326693)
  line L345 (114.290526, -122.326693) -> (117.636591, -123.223269)
  line L346 (117.636591, -123.223269) -> (118.533166, -126.569334)
  line L347 (118.533166, -126.569334) -> (116.083676, -129.018824)
  line L348 (116.083676, -129.018824) -> (112.737611, -128.122248)
  line L349 (112.737611, -128.122248) -> (111.841036, -124.776183)
  line L350 (119.112722, -126.414042) -> (118.216146, -123.067977)
  line L351 (118.216146, -123.067977) -> (120.665636, -120.618487)
  line L352 (120.665636, -120.618487) -> (124.011701, -121.515063)
  line L353 (124.011701, -121.515063) -> (124.908277, -124.861128)
  line L354 (124.908277, -124.861128) -> (122.458787, -127.310618)
  line L355 (122.458787, -127.310618) -> (119.112722, -126.414042)
  line L356 (123.779626, -131.080947) -> (122.883051, -127.734882)
  line L357 (122.883051, -127.734882) -> (125.332541, -125.285392)
  line L358 (125.332541, -125.285392) -> (128.678606, -126.181968)
  line L359 (128.678606, -126.181968) -> (129.575181, -129.528033)
  line L360 (129.575181, -129.528033) -> (127.125692, -131.977523)
  line L361 (127.125692, -131.977523) -> (123.779626, -131.080947)
  line L362 (133.500802, -130.269317) -> (130.154737, -129.372741)
  line L363 (130.154737, -129.372741) -> (129.258161, -126.026676)
  line L364 (129.258161, -126.026676) -> (131.707651, -123.577187)
  line L365 (131.707651, -123.577187) -> (135.053716, -124.473762)
  line L366 (135.053716, -124.473762) -> (135.950292, -127.819827)
  line L367 (135.950292, -127.819827) -> (133.500802, -130.269317)
  point P0 (0, 0)
  point P1 (87.978453, -138.880692)
  point P2 (92.232244, -135.051166)
  point P3 (91.455786, -137.948943)
  point P4 (96.474884, -139.293806)
  point P5 (97.251341, -136.396029)
  point P6 (90.524038, -141.426276)
  point P7 (89.747581, -144.324054)
  point P8 (94.766679, -145.668917)
  point P9 (95.543136, -142.771139)
  point P10 (96.899148, -139.71807)
  point P11 (96.122691, -142.615848)
  point P12 (101.141789, -143.960711)
  point P13 (101.918246, -141.062934)
  point P14 (101.566053, -144.384975)
  point P15 (100.789596, -147.282753)
  point P16 (105.808694, -148.627616)
  point P17 (106.585151, -145.729838)
  point P18 (107.516899, -142.252505)
  point P19 (108.293357, -139.354728)
  point P20 (103.274259, -138.009865)
  point P21 (102.497802, -140.907642)
  point P22 (107.941164, -142.676769)
  point P23 (107.164706, -145.574547)
  point P24 (112.183804, -146.91941)
  point P25 (112.960261, -144.021633)
  point P26 (112.608068, -147.343674)
  point P27 (111.831611, -150.241452)
  point P28 (116.850709, -151.586315)
  point P29 (117.627166, -148.688537)
  point P30 (118.558915, -145.211204)
  point P31 (119.335372, -142.313427)
  point P32 (114.316274, -140.968564)
  point P33 (113.539817, -143.866341)
  point P34 (118.983179, -145.635468)
  point P35 (118.206722, -148.533246)
  point P36 (123.225819, -149.878109)
  point P37 (124.002277, -146.980332)
  point P38 (123.650084, -150.302373)
  point P39 (122.873626, -153.200151)
  point P40 (127.892724, -154.545014)
  point P41 (128.669181, -151.647236)
  point P42 (129.60093, -148.169903)
  point P43 (130.377387, -145.272126)
  point P44 (125.358289, -143.927263)
  point P45 (124.581832, -146.82504)
  point P46 (86.788882, -133.282038)
  point P47 (87.565339, -130.384261)
  point P48 (92.584437, -131.729124)
  point P49 (91.80798, -134.626902)
  point P50 (93.940449, -128.676055)
  point P51 (93.163992, -131.573833)
  point P52 (98.18309, -132.918696)
  point P53 (98.959547, -130.020918)
  point P54 (98.607354, -133.34296)
  point P55 (97.830897, -136.240737)
  point P56 (102.849995, -137.585601)
  point P57 (103.626452, -134.687823)
  point P58 (104.206007, -134.532532)
  point P59 (104.982464, -131.634754)
  point P60 (110.001562, -132.979617)
  point P61 (109.225105, -135.877395)
  point P62 (109.649369, -136.301659)
  point P63 (114.668467, -137.646522)
  point P64 (113.89201, -140.5443)
  point P65 (108.872912, -139.199436)
  point P66 (115.248023, -137.491231)
  point P67 (116.02448, -134.593453)
  point P68 (121.043578, -135.938316)
  point P69 (120.26712, -138.836094)
  point P70 (119.914927, -142.158135)
  point P71 (120.691384, -139.260358)
  point P72 (125.710482, -140.605221)
  point P73 (124.934025, -143.502999)
  point P74 (126.290038, -140.44993)
  point P75 (127.066495, -137.552152)
  point P76 (132.085593, -138.897016)
  point P77 (131.309136, -141.794793)
  point P78 (88.497087, -126.906928)
  point P79 (89.273545, -124.00915)
  point P80 (94.292642, -125.354014)
  point P81 (93.516185, -128.251791)
  point P82 (95.648655, -122.300945)
  point P83 (94.872198, -125.198722)
  point P84 (99.891296, -126.543585)
  point P85 (100.667753, -123.645808)
  point P86 (100.31556, -126.967849)
  point P87 (99.539103, -129.865627)
  point P88 (104.5582, -131.21049)
  point P89 (105.334658, -128.312713)
  point P90 (105.914213, -128.157421)
  point P91 (106.69067, -125.259644)
  point P92 (111.709768, -126.604507)
  point P93 (110.933311, -129.502284)
  point P94 (111.357575, -129.926549)
  point P95 (116.376673, -131.271412)
  point P96 (115.600216, -134.169189)
  point P97 (110.581118, -132.824326)
  point P98 (116.956228, -131.11612)
  point P99 (117.732685, -128.218343)
  point P100 (122.751783, -129.563206)
  point P101 (121.975326, -132.460983)
  point P102 (121.623133, -135.783025)
  point P103 (122.39959, -132.885248)
  point P104 (127.418688, -134.230111)
  point P105 (126.642231, -137.127888)
  point P106 (127.998243, -134.074819)
  point P107 (128.774701, -131.177042)
  point P108 (133.793798, -132.521905)
  point P109 (133.017341, -135.419683)
  point P110 (88.391568, -147.377122)
  point P111 (89.168025, -144.479345)
  point P112 (84.148927, -143.134482)
  point P113 (83.37247, -146.032259)
  point P114 (88.815832, -147.801387)
  point P115 (93.83493, -149.14625)
  point P116 (93.058473, -152.044027)
  point P117 (88.039375, -150.699164)
  point P118 (99.857847, -150.760086)
  point P119 (99.08139, -153.657863)
  point P120 (99.433583, -150.335821)
  point P121 (94.414485, -148.990958)
  point P122 (95.190943, -146.093181)
  point P123 (100.21004, -147.438044)
  point P124 (104.876945, -152.104949)
  point P125 (104.100488, -155.002726)
  point P126 (105.456501, -151.949657)
  point P127 (106.232958, -149.05188)
  point P128 (111.252056, -150.396743)
  point P129 (110.475599, -153.294521)
  point P130 (110.899863, -153.718785)
  point P131 (110.123405, -156.616562)
  point P132 (115.142503, -157.961425)
  point P133 (115.91896, -155.063648)
  point P134 (121.517614, -156.25322)
  point P135 (117.274973, -152.010579)
  point P136 (116.498516, -154.908356)
  point P137 (122.294071, -153.355442)
  point P138 (121.941878, -156.677484)
  point P139 (126.960976, -158.022347)
  point P140 (126.184518, -160.920124)
  point P141 (121.165421, -159.575261)
  point P142 (86.683362, -153.752233)
  point P143 (87.45982, -150.854455)
  point P144 (82.440722, -149.509592)
  point P145 (81.664265, -152.40737)
  point P146 (87.107626, -154.176497)
  point P147 (92.126724, -155.52136)
  point P148 (91.350267, -158.419138)
  point P149 (86.331169, -157.074274)
  point P150 (98.149642, -157.135196)
  point P151 (97.373185, -160.032973)
  point P152 (97.725378, -156.710932)
  point P153 (92.70628, -155.366069)
  point P154 (93.482737, -152.468291)
  point P155 (98.501835, -153.813154)
  point P156 (103.16874, -158.480059)
  point P157 (102.392282, -161.377837)
  point P158 (103.748295, -158.324768)
  point P159 (104.524752, -155.42699)
  point P160 (109.54385, -156.771854)
  point P161 (108.767393, -159.669631)
  point P162 (109.191657, -160.093895)
  point P163 (108.4152, -162.991673)
  point P164 (113.434298, -164.336536)
  point P165 (114.210755, -161.438758)
  point P166 (119.809408, -162.62833)
  point P167 (115.566767, -158.385689)
  point P168 (114.79031, -161.283467)
  point P169 (120.585865, -159.730553)
  point P170 (120.233672, -163.052594)
  point P171 (125.25277, -164.397457)
  point P172 (124.476313, -167.295235)
  point P173 (119.457215, -165.950372)
  point P174 (84.975157, -160.127343)
  point P175 (85.751614, -157.229566)
  point P176 (80.732516, -155.884703)
  point P177 (79.956059, -158.78248)
  point P178 (85.399421, -160.551607)
  point P179 (90.418519, -161.896471)
  point P180 (89.642061, -164.794248)
  point P181 (84.622964, -163.449385)
  point P182 (96.441436, -163.510306)
  point P183 (95.664979, -166.408084)
  point P184 (96.017172, -163.086042)
  point P185 (90.998074, -161.741179)
  point P186 (91.774531, -158.843402)
  point P187 (96.793629, -160.188265)
  point P188 (101.460534, -164.85517)
  point P189 (100.684077, -167.752947)
  point P190 (102.040089, -164.699878)
  point P191 (102.816546, -161.802101)
  point P192 (107.835644, -163.146964)
  point P193 (107.059187, -166.044741)
  point P194 (107.483451, -166.469006)
  point P195 (106.706994, -169.366783)
  point P196 (111.726092, -170.711646)
  point P197 (112.502549, -167.813869)
  point P198 (118.101202, -169.003441)
  point P199 (113.858562, -164.7608)
  dimension "d1" = 6.5
  dimension "d2" = 7
  dimension "d6" = 12
  dimension "d57" = 20